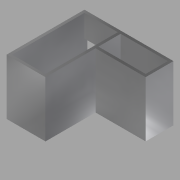
# Autodesk Inventor part: RSX Structure
Saved by Autodesk Inventor 2017 (Build 210142000, 142)
## iProperties
Created: 2016-10-27
Part Number: RSX Structure
Material: Aluminum 6061
Document SubType Name: Modeling
Designer: eschr_000
Density: 2.7 g/cm^3
Appearance: Aluminum - Flat
Mass: 208.831 g
Surface Area: 3384.58 cm^2
Volume: 77.3448 cm^3
Author: eschr_000
Autodesk Inventor part; units mm, degrees
ref_plane "YZ Plane" through (0, 0, 0) normal (1, 0, 0) x (0, 1, 0)
ref_plane "XZ Plane" through (0, 0, 0) normal (0, 1, 0) x (-1, 0, 0)
ref_plane "XY Plane" through (0, 0, 0) normal (0, 0, 1) x (1, 0, 0)
sketch "Sketch2" plane through (0, 0, 0) normal (0, 1, 0) x (-1, 0, 0)
  line L0 (0, 0) -> (177.8, 0)
  line L1 (177.8, 0) -> (177.8, -203.2)
  line L2 (177.8, -203.2) -> (0, -203.2)
  line L3 (0, -203.2) -> (0, 0)
  dimension "d0" = 203.2
  dimension "d1" = 177.8
  constraints: 8 end point, 2 parallel, 1 horizontal, 1 perpendicular
  measures "d0" distance of L2.end L0.start
  measures "d1" distance of L1.end L2.end
extrude "Extrusion1" add sketch "Sketch2" along normal blind 12.7
sketch "Sketch3" plane through (0, 12.7, 0) normal (0, 1, 0) x (1, 0, 0)
  line L0 (0, 0) -> (-177.8, 0)
  line L1 (-177.8, 0) -> (-177.8, 203.2)
  line L2 (-177.8, 203.2) -> (0, 203.2)
  line L3 (0, 203.2) -> (0, 0)
  line L4 (-171.45, 196.85) -> (-171.45, 6.35)
  line L5 (-171.45, 6.35) -> (-6.35, 6.35)
  line L6 (-6.35, 6.35) -> (-6.35, 196.85)
  line L7 (-6.35, 196.85) -> (-171.45, 196.85)
  dimension "d4" = 6.35
  constraints: 16 end point, 4 parallel, 2 perpendicular, 1 horizontal, 3 other
  measures "d4" distance between parallel lines of L1 L4
extrude "Extrusion2" add sketch "Sketch3" along normal blind 114.3
sketch "Sketch5" plane through (0, 12.7, 0) normal (0, 1, 0) x (1, 0, 0)
  line L0 (-63.5, 114.3) -> (-63.5, 6.35)
  line L1 (-6.35, 120.65) -> (-6.3512, 120.1928)
  line L2 (-171.45, 114.3) -> (-63.5, 114.3)
  line L3 (-171.45, 6.35) -> (-171.45, 196.85) projected
  line L4 (-6.35, 6.35) -> (-171.45, 6.35) projected
  line L5 (-171.45, 120.65) -> (-57.15, 120.65)
  line L6 (-57.15, 114.3) -> (-57.15, 6.35)
  line L7 (-171.45, 120.65) -> (-6.35, 120.65)
  line L8 (-57.15, 114.3) -> (-6.35, 114.3)
  line L9 (-6.35, 196.85) -> (-6.35, 6.35) projected
  line L10 (-171.45, 120.65) -> (-171.45, 114.3)
  line L11 (-6.35, 120.65) -> (-6.35, 114.3)
  line L12 (-6.35, 120.65) -> (-6.35, 114.3)
  line L13 (-63.5, 6.35) -> (-57.15, 6.35)
  line L14 (-171.45, 6.35) -> (-6.35, 6.35) projected
  dimension "d36" = 107.95
  dimension "d37" = 107.95
  dimension "d38" = 6.35
  constraints: 22 end point, 4 collinear, 2 horizontal, 1 parallel, 1 point on line
  measures "d36" distance between parallel lines of L0 L3
  measures "d37" distance between parallel lines of L2 L4
  measures "d38" distance between parallel lines of L2 L5
extrude "Extrusion5" add sketch "Sketch5" along normal blind 114.3 contours L2 L3 L5 L7 L1 L9 L8 L6 L4 L0
sketch "Sketch6" plane through (0, 0, 0) normal (0, -1, 0) x (1, 0, 0)
  line L0 (0, -203.2) -> (-177.8, 0) construction
  circle A0 centre (-88.9, -101.6) radius 101.6 construction
  line L1 (-177.8, -203.2) -> (0, 0) construction
  point P0 (-155.8041, -178.0618)
  point P1 (-155.8041, -25.1382)
  point P2 (-21.9959, -25.1382)
  point P3 (-21.9959, -178.0618)
  dimension "d25" = 203.2
  constraints: 4 end point, 4 point on circle, 4 point on line, 1 centre point, 1 coincident, 1 midpoint
  measures "d25" diameter of A0
hole "Hole1" at (-21.9959, 0, -25.1382) at (-155.8041, 0, -25.1382) at (-155.8041, 0, -178.0618) at (-21.9959, 0, -178.0618) direction (0, 1, 0) diameter 9.8044 end through all
sketch "Sketch7" plane through (-6.35, 12.7, -196.85) normal (-1, 0, 0) x (0, 0, 1)
  line L0 (76.2, 0) -> (0, 0) projected
  line L1 (76.2, 0) -> (76.2, 114.3) projected
  line L2 (0, 0) -> (76.2, 0)
  line L3 (76.2, 0) -> (76.2, 63.5)
  line L4 (76.2, 63.5) -> (0, 63.5)
  line L5 (0, 63.5) -> (0, 0)
  point P0 (196.85, -12.7)
  dimension "d39" = 63.5
  constraints: 8 end point, 2 parallel, 1 horizontal, 1 perpendicular, 1 point on line
  measures "d39" distance of L4.end L0.end
extrude "Extrusion6" cut sketch "Sketch7" against normal blind 6.35
sketch "Sketch8" plane through (-177.8, 0, -203.2) normal (-1, 0, 0) x (0, 0, 1)
  line L0 (88.9, 12.7) -> (88.9, 127) projected
  line L1 (196.85, 127) -> (88.9, 127) projected
  line L2 (196.85, 12.7) -> (196.85, 127) projected
  line L3 (88.9, 12.7) -> (196.85, 12.7) projected
  point P0 (203.2, 0)
extrude "Extrusion7" cut sketch "Sketch8" against normal up to surface (114.3 mm away)
sketch "Sketch9" plane through (-177.8, 0, 0) normal (0, 0, 1) x (1, 0, 0)
  line L0 (0, 12.7) -> (114.3, 12.7) projected
  line L1 (114.3, 12.7) -> (114.3, 127) projected
  line L2 (0, 127) -> (114.3, 127) projected
  line L3 (0, 12.7) -> (0, 127) projected
  point P0 (177.8, 0)
extrude "Extrusion8" cut sketch "Sketch9" against normal up to surface (114.3 mm away)
sketch "Sketch10" plane through (0, 12.7, 0) normal (0, 1, 0) x (1, 0, 0)
  circle A0 centre (-155.8041, 25.1382) radius 4.9022 projected
  line L0 (-177.8, 114.3) -> (-63.5, 114.3) projected
  line L1 (-177.8, 0) -> (-177.8, 114.3) projected
  line L2 (-63.5, 0) -> (-177.8, 0) projected
  line L3 (-63.5, 0) -> (-63.5, 114.3) projected
  line L4 (-177.8, 0) -> (-177.8, 114.3) projected
  line L5 (-6.35, 114.3) -> (-6.35, 6.35) projected
  line L6 (-6.35, 6.35) -> (-57.15, 6.35) projected
  line L7 (-57.15, 6.35) -> (-57.15, 114.3) projected
  line L8 (-57.15, 114.3) -> (-6.35, 114.3) projected
  line L9 (-171.45, 120.65) -> (-171.45, 196.85) projected
  line L10 (-171.45, 196.85) -> (-6.35, 196.85) projected
  line L11 (-6.35, 196.85) -> (-6.35, 120.65) projected
  line L12 (-6.35, 120.65) -> (-171.45, 120.65) projected
  line L13 (-63.5, 114.3) -> (-63.5, 0) projected
  line L14 (-63.5, 0) -> (0, 0) projected
  line L15 (0, 0) -> (0, 203.2) projected
  line L16 (0, 203.2) -> (-177.8, 203.2) projected
  line L17 (-177.8, 203.2) -> (-177.8, 114.3) projected
  line L18 (-177.8, 114.3) -> (-63.5, 114.3) projected
  point P0 (-177.8, 66.675)
  constraints: 1 point on line
extrude "Extrusion10" cut sketch "Sketch10" against normal through all contours L0 L3 L2 L1
body "Solid1"
